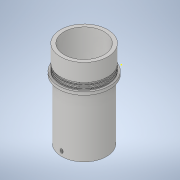
# Autodesk Inventor part: akkufach
Saved by Autodesk Inventor 2022 (Build 260153000, 153)
## iProperties
Created: 2019-01-21
Part Number: akkufach
Material: Generisch
Document SubType Name: Modeling
Designer: g.schardt
Density: 1 g/cm^3
Appearance: Vorgabe
Author: g.schardt
Autodesk Inventor part; units mm, degrees
sketch "Skizze1" plane through (0, 0, 0) normal (0, 0, 1) x (1, 0, 0)
  circle A0 centre (0, 0) radius 24.4
  dimension "d0" = 48.8
  constraints: 1 centre point, 1 coincident
  measures "d0" diameter of A0
extrude "Extrusion1" add sketch "Skizze1" against normal blind 90
sketch "Skizze5" plane through (0, 0, 0) normal (0, 0, 1) x (1, 0, 0)
  circle A0 centre (0, 0) radius 21.5
  dimension "d21" = 43
  constraints: 1 centre point, 1 coincident
  measures "d21" diameter of A0
extrude "Extrusion2" [suppressed]
ref_plane "Arbeitsebene1" through (0, 0, -25) normal (0, 0, -1) x (-1, 0, 0)
sketch "Skizze6" plane through (0, 0, -25) normal (0, 0, -1) x (-1, 0, 0)
  circle A0 centre (0, 0) radius 26.5
  dimension "d25" = 53
  constraints: 1 centre point, 1 coincident
  measures "d25" diameter of A0
extrude "Extrusion3" add sketch "Skizze6" along normal blind 3
ref_plane "Arbeitsebene2" through (0, 0, -24) normal (0, 0, 1) x (1, 0, 0)
sketch "Skizze7" plane through (0, 0, -24) normal (0, 0, 1) x (1, 0, 0)
  circle A0 centre (0, 0) radius 23.2
  circle A1 centre (0, 0) radius 24.4
  dimension "d29" = 46.4
  constraints: 2 centre point, 2 coincident
  measures "d29" diameter of A0
extrude "Extrusion4" cut sketch "Skizze7" along normal blind 2.2
ref_plane "Arbeitsebene3" through (0, 0, -20.4) normal (0, 0, 1) x (1, 0, 0)
sketch "Skizze8" plane through (0, 0, -20.4) normal (0, 0, 1) x (1, 0, 0)
  circle A0 centre (0, 0) radius 23.2
  circle A1 centre (0, 0) radius 24.4
  dimension "d33" = 46.4
  constraints: 2 centre point, 2 coincident
  measures "d33" diameter of A0
extrude "Extrusion5" cut sketch "Skizze8" along normal blind 2.2
fillet "Rundung1" radius 0.2 4 edges at (-24.4, 0, -24) (-24.4, 0, -21.8) (-24.4, 0, -20.4) (-24.4, 0, -18.2)
fillet "Rundung2" radius 0.3 4 edges at (-23.2, 0, -24) (-23.2, 0, -20.4) (-23.2, 0, -18.2) (-23.2, 0, -21.8)
sketch "Skizze3" plane through (0, 0, 0) normal (0, 0, 1) x (1, 0, 0)
  point P0 (0, 0)
  point P1 (0, 0)
  constraints: 1 coincident
hole "Bohrung2" at (0, 0, 0) direction (0, 0, -1) diameter 41.4 depth 80
sketch "Skizze14" plane through (0, 0, -90) normal (0, 0, -1) x (-1, 0, 0)
  point P0 (0, 0)
  point P1 (0, 0)
  constraints: 1 coincident
hole "Bohrung4" at (0, 0, -90) direction (0, 0, 1) diameter 16.2 depth 10
chamfer "Fase2" distance 0.5 angle 45 1 edges at (0, -8.1, -90)
sketch "Skizze15" plane through (0, 0, -80) normal (0, 0, 1) x (1, 0, 0)
  point P0 (0, 0)
  point P1 (0, 0)
  constraints: 1 coincident
hole "Bohrung5" at (0, 0, -80) direction (0, 0, -1) diameter 30 depth 5
sketch "Skizze16" plane through (0, 0, 0) normal (1, 0, 0) x (0, 1, 0)
  line L0 (-28.5003, -80.2428) -> (-15.6915, -93.0517)
  line L1 (-28.5003, -80.2428) -> (-10.3858, -80.2428) construction
  line L2 (-24.4, -28) -> (-24.4, -90) projected
  line L3 (-24.4, -90) -> (24.4, -90) projected
  point P0 (0, 0)
  dimension "d75" = 45
  dimension "d83" = 4
  constraints: 4 end point, 1 equal length, 1 horizontal
  measures "d75" angle of L0 L1
  measures "d83" distance from line of L2.end L0
ref_plane "Arbeitsebene7" through (0, 0, -10) normal (-1, 0, 0) x (0, 0, 1)
ref_plane "Arbeitsebene9" through (0, -15.6915, -93.0517) normal (0, 0.7071, -0.7071) x (-1, 0, 0)
sketch "Skizze17" plane through (0, -15.6915, -93.0517) normal (0, 0.7071, -0.7071) x (-1, 0, 0)
  point P0 (0, 76.893)
sketch "Skizze18" plane through (0, -15.6915, -93.0517) normal (0, 0.7071, -0.7071) x (-1, 0, 0)
  point P0 (0, 76.893)
  point P1 (0, 0.393)
  dimension "d91" = 76.5
  constraints: 1 vertical alignment
  measures "d91" distance of point (0, 0.393) point (0, 76.893)
hole "Bohrung6" at (0, -15.4136, -92.7738) direction (0, -0.7071, 0.7071) diameter 3 end through all
sketch "Skizze19" plane through (0, 0, -90) normal (0, 0, -1) x (-1, 0, 0)
  circle A0 centre (0, 0) radius 23.25
  circle A1 centre (0, 0) radius 24.4 projected
  dimension "d84" = 46.5
  constraints: 1 centre point, 1 coincident
  measures "d84" diameter of A0
extrude "Extrusion8" cut sketch "Skizze19" against normal up to surface (62 mm away)
sketch "Skizze20" plane through (0, 0, -3) normal (0, 0, 1) x (1, 0, 0)
  circle A0 centre (0, 0) radius 21.75
  dimension "d88" = 43.5
  constraints: 1 centre point, 1 coincident
  measures "d88" diameter of A0
